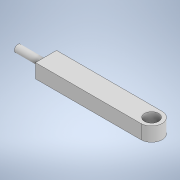
# Autodesk Inventor part: Arm
Saved by Autodesk Inventor 2021 (Build 250183000, 183)
## iProperties
Created: 2022-10-04
Part Number: Arm
Material: Generic
Document SubType Name: Modeling
Designer: mrizw
Density: 1 g/cm^3
Appearance: Default
Author: mrizw
Autodesk Inventor part; units mm, degrees
ref_plane "YZ Plane" through (0, 0, 0) normal (1, 0, 0) x (0, 1, 0)
ref_plane "XZ Plane" through (0, 0, 0) normal (0, 1, 0) x (-1, 0, 0)
ref_plane "XY Plane" through (0, 0, 0) normal (0, 0, 1) x (1, 0, 0)
sketch "Sketch1" plane through (0, 0, 0) normal (0, 1, 0) x (-1, 0, 0)
  point P0 (0, 0)
sketch "Sketch2" plane through (0, 0, 0) normal (0, 1, 0) x (-1, 0, 0)
  line L0 (0, 0) -> (0, -7.5)
  line L1 (0, -7.5) -> (75, -7.5)
  line L2 (75, -7.5) -> (75, 7.5)
  line L3 (75, 7.5) -> (0, 7.5)
  line L4 (0, 7.5) -> (0, 0)
  arc A0 (0, 7.5) -> (0, -7.5) centre (0, 0) ccw
  dimension "d0" = 7.5
  dimension "d1" = 75
  dimension "d2" = 15
  constraints: 10 end point, 2 perpendicular, 2 point on circle, 1 centre point, 1 horizontal, 1 tangent, 1 vertical
  measures "d0" distance of L0.start L0.end
  measures "d1" distance of L0.end L1.end
  measures "d2" distance of L1.end L2.end
extrude "Extrusion1" add sketch "Sketch2" along normal blind 10
sketch "Sketch3" plane through (0, 10, 0) normal (0, 1, 0) x (1, 0, 0)
  point P0 (0, 0)
  point P1 (0, 0)
  constraints: 1 coincident
hole "Hole1" at (0, 10, 0) direction (0, -1, 0) diameter 10 end through all
sketch "Sketch4" plane through (-75, 0, -7.5) normal (-1, 0, 0) x (0, 0, 1)
  circle A0 centre (7.5, 5) radius 2.5
  point P0 (7.5, 0)
  dimension "d14" = 5
  constraints: 1 centre point
  measures "d14" diameter of A0
extrude "Extrusion2" add sketch "Sketch4" along normal blind 20
body "Solid1"
